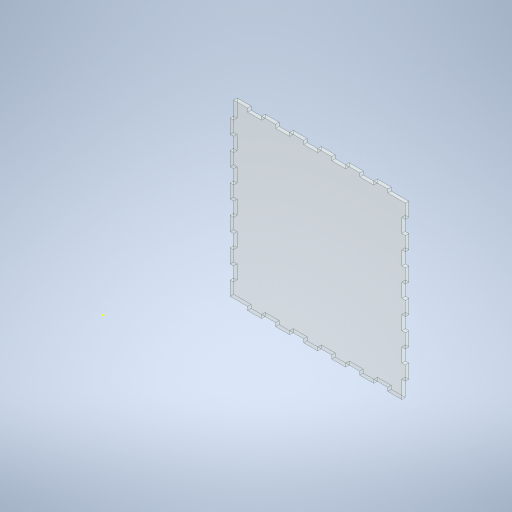
# Autodesk Inventor part: Part1
Saved by Autodesk Inventor 2024 (Build 280153000, 153)
## iProperties
Created: 2023-10-19
Part Number: Part1
Material: Glass
Document SubType Name: Modeling
Designer: liuyu
Density: 2.18 g/cm^3
Appearance: Clear
Author: liuyu
Autodesk Inventor part; units mm, degrees
ref_plane "YZ Plane" through (0, 0, 0) normal (1, 0, 0) x (0, 1, 0)
ref_plane "XZ Plane" through (0, 0, 0) normal (0, 1, 0) x (-1, 0, 0)
ref_plane "XY Plane" through (0, 0, 0) normal (0, 0, 1) x (1, 0, 0)
sketch "Sketch1" plane through (0, 0, 0) normal (0, 0, 1) x (1, 0, 0)
  line L0 (425.9934, 353.49) -> (405.9934, 353.49)
  line L1 (185.9934, 353.49) -> (185.9934, 358.49)
  line L2 (185.9934, 358.49) -> (205.9934, 358.49)
  line L3 (205.9934, 358.49) -> (205.9934, 353.49)
  line L4 (225.9934, 353.49) -> (225.9934, 358.49)
  line L5 (225.9934, 358.49) -> (245.9934, 358.49)
  line L6 (245.9934, 358.49) -> (245.9934, 353.49)
  line L7 (265.9934, 353.49) -> (265.9934, 358.49)
  line L8 (265.9934, 358.49) -> (285.9934, 358.49)
  line L9 (285.9934, 358.49) -> (285.9934, 353.49)
  line L10 (305.9934, 353.49) -> (305.9934, 358.49)
  line L11 (305.9934, 358.49) -> (325.9934, 358.49)
  line L12 (325.9934, 358.49) -> (325.9934, 353.49)
  line L13 (345.9934, 353.49) -> (345.9934, 358.49)
  line L14 (345.9934, 358.49) -> (365.9934, 358.49)
  line L15 (365.9934, 358.49) -> (365.9934, 353.49)
  line L16 (385.9934, 353.49) -> (385.9934, 358.49)
  line L17 (385.9934, 358.49) -> (405.9934, 358.49)
  line L18 (405.9934, 358.49) -> (405.9934, 353.49)
  line L19 (385.9934, 353.49) -> (365.9934, 353.49)
  line L20 (345.9934, 353.49) -> (325.9934, 353.49)
  line L21 (305.9934, 353.49) -> (285.9934, 353.49)
  line L22 (265.9934, 353.49) -> (245.9934, 353.49)
  line L23 (225.9934, 353.49) -> (205.9934, 353.49)
  line L24 (425.9934, 113.49) -> (425.9934, 133.49)
  line L25 (425.9934, 353.49) -> (430.9934, 353.49)
  line L26 (430.9934, 353.49) -> (430.9934, 333.49)
  line L27 (430.9934, 333.49) -> (425.9934, 333.49)
  line L28 (425.9934, 313.49) -> (430.9934, 313.49)
  line L29 (430.9934, 313.49) -> (430.9934, 293.49)
  line L30 (430.9934, 293.49) -> (425.9934, 293.49)
  line L31 (425.9934, 273.49) -> (430.9934, 273.49)
  line L32 (430.9934, 273.49) -> (430.9934, 253.49)
  line L33 (430.9934, 253.49) -> (425.9934, 253.49)
  line L34 (425.9934, 233.49) -> (430.9934, 233.49)
  line L35 (430.9934, 233.49) -> (430.9934, 213.49)
  line L36 (430.9934, 213.49) -> (425.9934, 213.49)
  line L37 (425.9934, 193.49) -> (430.9934, 193.49)
  line L38 (430.9934, 193.49) -> (430.9934, 173.49)
  line L39 (430.9934, 173.49) -> (425.9934, 173.49)
  line L40 (425.9934, 153.49) -> (430.9934, 153.49)
  line L41 (430.9934, 153.49) -> (430.9934, 133.49)
  line L42 (430.9934, 133.49) -> (425.9934, 133.49)
  line L43 (425.9934, 153.49) -> (425.9934, 173.49)
  line L44 (425.9934, 193.49) -> (425.9934, 213.49)
  line L45 (425.9934, 233.49) -> (425.9934, 253.49)
  line L46 (425.9934, 273.49) -> (425.9934, 293.49)
  line L47 (425.9934, 313.49) -> (425.9934, 333.49)
  line L48 (185.9934, 353.49) -> (185.9934, 333.49)
  line L49 (185.9934, 113.49) -> (180.9934, 113.49)
  line L50 (180.9934, 113.49) -> (180.9934, 133.49)
  line L51 (180.9934, 133.49) -> (185.9934, 133.49)
  line L52 (185.9934, 153.49) -> (180.9934, 153.49)
  line L53 (180.9934, 153.49) -> (180.9934, 173.49)
  line L54 (180.9934, 173.49) -> (185.9934, 173.49)
  line L55 (185.9934, 193.49) -> (180.9934, 193.49)
  line L56 (180.9934, 193.49) -> (180.9934, 213.49)
  line L57 (180.9934, 213.49) -> (185.9934, 213.49)
  line L58 (185.9934, 233.49) -> (180.9934, 233.49)
  line L59 (180.9934, 233.49) -> (180.9934, 253.49)
  line L60 (180.9934, 253.49) -> (185.9934, 253.49)
  line L61 (185.9934, 273.49) -> (180.9934, 273.49)
  line L62 (180.9934, 273.49) -> (180.9934, 293.49)
  line L63 (180.9934, 293.49) -> (185.9934, 293.49)
  line L64 (185.9934, 313.49) -> (180.9934, 313.49)
  line L65 (180.9934, 313.49) -> (180.9934, 333.49)
  line L66 (180.9934, 333.49) -> (185.9934, 333.49)
  line L67 (185.9934, 313.49) -> (185.9934, 293.49)
  line L68 (185.9934, 273.49) -> (185.9934, 253.49)
  line L69 (185.9934, 233.49) -> (185.9934, 213.49)
  line L70 (185.9934, 193.49) -> (185.9934, 173.49)
  line L71 (185.9934, 153.49) -> (185.9934, 133.49)
  line L72 (185.9934, 113.49) -> (205.9934, 113.49)
  line L73 (425.9934, 113.49) -> (425.9934, 108.49)
  line L74 (425.9934, 108.49) -> (405.9934, 108.49)
  line L75 (405.9934, 108.49) -> (405.9934, 113.49)
  line L76 (385.9934, 113.49) -> (385.9934, 108.49)
  line L77 (385.9934, 108.49) -> (365.9934, 108.49)
  line L78 (365.9934, 108.49) -> (365.9934, 113.49)
  line L79 (345.9934, 113.49) -> (345.9934, 108.49)
  line L80 (345.9934, 108.49) -> (325.9934, 108.49)
  line L81 (325.9934, 108.49) -> (325.9934, 113.49)
  line L82 (305.9934, 113.49) -> (305.9934, 108.49)
  line L83 (305.9934, 108.49) -> (285.9934, 108.49)
  line L84 (285.9934, 108.49) -> (285.9934, 113.49)
  line L85 (265.9934, 113.49) -> (265.9934, 108.49)
  line L86 (265.9934, 108.49) -> (245.9934, 108.49)
  line L87 (245.9934, 108.49) -> (245.9934, 113.49)
  line L88 (225.9934, 113.49) -> (225.9934, 108.49)
  line L89 (225.9934, 108.49) -> (205.9934, 108.49)
  line L90 (205.9934, 108.49) -> (205.9934, 113.49)
  line L91 (225.9934, 113.49) -> (245.9934, 113.49)
  line L92 (265.9934, 113.49) -> (285.9934, 113.49)
  line L93 (305.9934, 113.49) -> (325.9934, 113.49)
  line L94 (345.9934, 113.49) -> (365.9934, 113.49)
  line L95 (385.9934, 113.49) -> (405.9934, 113.49)
  point P0 (0, 0)
  constraints: 192 end point
extrude "Extrusion1" add sketch "Sketch1" along normal blind 5
sketch "Sketch2" plane through (0, 0, 5) normal (0, 0, 1) x (1, 0, 0)
  point P0 (0, 0)
body "Solid1"
